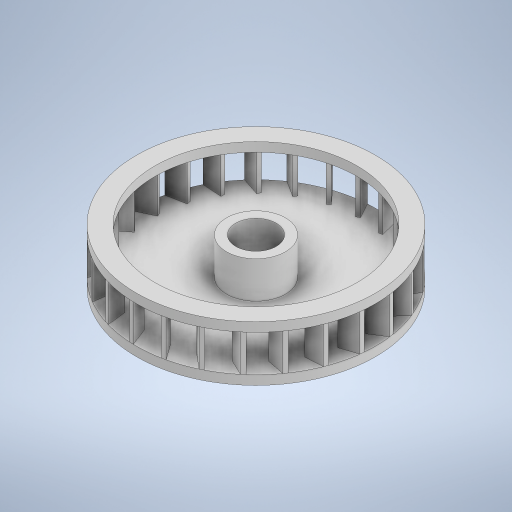
# Autodesk Inventor part: taiya1
Saved by Autodesk Inventor 2023.2 (Build 272271000, 271)
## iProperties
Created: 2022-12-08
Part Number: taiya1
Material: 一般
Document SubType Name: Modeling
Designer: 千葉 俊輔
Density: 1 g/cm^3
Appearance: 既定
Author: 千葉 俊輔
Autodesk Inventor part; units mm, degrees
ref_plane "YZ Plane" through (0, 0, 0) normal (1, 0, 0) x (0, 1, 0)
ref_plane "XZ Plane" through (0, 0, 0) normal (0, 1, 0) x (-1, 0, 0)
ref_plane "XY Plane" through (0, 0, 0) normal (0, 0, 1) x (1, 0, 0)
sketch "スケッチ1" plane through (0, 0, 0) normal (0, 1, 0) x (-1, 0, 0)
  circle A0 centre (0, 0) radius 65
  dimension "d0" = 130
  constraints: 1 centre point, 1 coincident
  measures "d0" diameter of A0
extrude "押し出し1" add sketch "スケッチ1" along normal blind 5
sketch "スケッチ2" plane through (0, 5, 0) normal (0, 1, 0) x (1, 0, 0)
  circle A0 centre (0, 0) radius 65 projected
  line L0 (-64.9999, -0.1391) -> (-56.3899, 3.8758)
  line L1 (-56.3899, 3.8758) -> (-55.5447, 2.0632)
  line L2 (-55.5447, 2.0632) -> (-64.1546, -1.9517)
  line L3 (-64.1546, -1.9517) -> (-64.9999, -0.1391)
  line L4 (-64.9999, -0.1391) -> (-55.4999, -0.1391) construction
  line L5 (-64.1546, -1.9517) -> (-64.9584, -2.3265)
  line L6 (-64.9999, -0.1391) -> (-64.9584, -2.3265)
  dimension "d4" = 25
  dimension "d5" = 9.5
  dimension "d6" = 2
  constraints: 14 end point, 2 parallel, 2 perpendicular, 2 point on circle, 1 equal length, 1 horizontal
  measures "d4" angle of L4 L0
  measures "d5" distance of L0.end L0.start
  measures "d6" distance of L2.end L0.start
extrude "押し出し2" add sketch "スケッチ2" along normal blind 20 contours L0 L1 L2 L3 | L3 L5 L6
pattern_circular "円形状パターン1" count 25 over 360 about axis through (0, 0, 0) along (0, 1, 0) of "押し出し2"
sketch "スケッチ6" plane through (0, 5, 0) normal (0, 1, 0) x (1, 0, 0)
  circle A0 centre (0, 0) radius 16
  circle A1 centre (0, 0) radius 11
  dimension "d14" = 32
  dimension "d15" = 22
  constraints: 2 centre point, 2 coincident
  measures "d14" diameter of A0
  measures "d15" diameter of A1
extrude "押し出し3" add sketch "スケッチ6" along normal blind 20
sketch "スケッチ7" plane through (0, 25, 0) normal (0, 1, 0) x (1, 0, 0)
  circle A0 centre (0, 0) radius 11 projected
  circle A1 centre (0, 0) radius 65
  circle A2 centre (0, 0) radius 55
  dimension "d18" = 130
  dimension "d19" = 110
  constraints: 2 centre point, 2 coincident
  measures "d18" diameter of A1
  measures "d19" diameter of A2
extrude "押し出し4" add sketch "スケッチ7" along normal blind 5 contours A1
